Autodesk Fusion 360 part; units mm, degrees
(part 9 of 9)
  line L507 (94.532, 88.6913) -> (90.2019, 91.1913)
  line L508 (100.3622, 91.1913) -> (96.032, 88.6913)
  line L509 (96.032, 88.6913) -> (96.032, 83.6913)
  line L510 (96.032, 83.6913) -> (100.3622, 81.1913)
  line L511 (100.3622, 81.1913) -> (104.6923, 83.6913)
  line L512 (104.6923, 83.6913) -> (104.6923, 88.6913)
  line L513 (104.6923, 88.6913) -> (100.3622, 91.1913)
  line L514 (14, 99.9904) -> (9.6699, 97.4904)
  line L515 (9.6699, 97.4904) -> (9.6699, 92.4904)
  line L516 (9.6699, 92.4904) -> (14, 89.9904)
  line L517 (14, 89.9904) -> (18.3301, 92.4904)
  line L518 (18.3301, 92.4904) -> (18.3301, 97.4904)
  line L519 (18.3301, 97.4904) -> (14, 99.9904)
  line L520 (24.1603, 99.9904) -> (19.8301, 97.4904)
  line L521 (19.8301, 97.4904) -> (19.8301, 92.4904)
  line L522 (19.8301, 92.4904) -> (24.1603, 89.9904)
  line L523 (24.1603, 89.9904) -> (28.4904, 92.4904)
  line L524 (28.4904, 92.4904) -> (28.4904, 97.4904)
  line L525 (28.4904, 97.4904) -> (24.1603, 99.9904)
  line L526 (34.3205, 99.9904) -> (29.9904, 97.4904)
  line L527 (29.9904, 97.4904) -> (29.9904, 92.4904)
  line L528 (29.9904, 92.4904) -> (34.3205, 89.9904)
  line L529 (34.3205, 89.9904) -> (38.6506, 92.4904)
  line L530 (38.6506, 92.4904) -> (38.6506, 97.4904)
  line L531 (38.6506, 97.4904) -> (34.3205, 99.9904)
  line L532 (44.4808, 99.9904) -> (40.1506, 97.4904)
  line L533 (40.1506, 97.4904) -> (40.1506, 92.4904)
  line L534 (40.1506, 92.4904) -> (44.4808, 89.9904)
  line L535 (44.4808, 89.9904) -> (48.8109, 92.4904)
  line L536 (48.8109, 92.4904) -> (48.8109, 97.4904)
  line L537 (48.8109, 97.4904) -> (44.4808, 99.9904)
  line L538 (54.641, 99.9904) -> (50.3109, 97.4904)
  line L539 (50.3109, 97.4904) -> (50.3109, 92.4904)
  line L540 (50.3109, 92.4904) -> (54.641, 89.9904)
  line L541 (54.641, 89.9904) -> (58.9711, 92.4904)
  line L542 (58.9711, 92.4904) -> (58.9711, 97.4904)
  line L543 (58.9711, 97.4904) -> (54.641, 99.9904)
  line L544 (64.8013, 99.9904) -> (60.4711, 97.4904)
  line L545 (60.4711, 97.4904) -> (60.4711, 92.4904)
  line L546 (60.4711, 92.4904) -> (64.8013, 89.9904)
  line L547 (64.8013, 89.9904) -> (69.1314, 92.4904)
  line L548 (69.1314, 92.4904) -> (69.1314, 97.4904)
  line L549 (69.1314, 97.4904) -> (64.8013, 99.9904)
  line L550 (74.9615, 99.9904) -> (70.6314, 97.4904)
  line L551 (70.6314, 97.4904) -> (70.6314, 92.4904)
  line L552 (70.6314, 92.4904) -> (74.9615, 89.9904)
  line L553 (74.9615, 89.9904) -> (79.2916, 92.4904)
  line L554 (79.2916, 92.4904) -> (79.2916, 97.4904)
  line L555 (79.2916, 97.4904) -> (74.9615, 99.9904)
  line L556 (85.1218, 99.9904) -> (80.7916, 97.4904)
  line L557 (80.7916, 97.4904) -> (80.7916, 92.4904)
  line L558 (80.7916, 92.4904) -> (85.1218, 89.9904)
  line L559 (85.1218, 89.9904) -> (89.4519, 92.4904)
  line L560 (89.4519, 92.4904) -> (89.4519, 97.4904)
  line L561 (89.4519, 97.4904) -> (85.1218, 99.9904)
  line L562 (95.282, 99.9904) -> (90.9519, 97.4904)
  line L563 (90.9519, 97.4904) -> (90.9519, 92.4904)
  line L564 (90.9519, 92.4904) -> (95.282, 89.9904)
  line L565 (95.282, 89.9904) -> (99.6122, 92.4904)
  line L566 (99.6122, 92.4904) -> (99.6122, 97.4904)
  line L567 (99.6122, 97.4904) -> (95.282, 99.9904)
  line L568 (105.4423, 99.9904) -> (101.1122, 97.4904)
  line L569 (101.1122, 97.4904) -> (101.1122, 92.4904)
  line L570 (101.1122, 92.4904) -> (105.4423, 89.9904)
  line L571 (105.4423, 89.9904) -> (109.7724, 92.4904)
  line L572 (109.7724, 92.4904) -> (109.7724, 97.4904)
  line L573 (109.7724, 97.4904) -> (105.4423, 99.9904)
  line L574 (19.0801, 108.7894) -> (14.75, 106.2894)
  line L575 (14.75, 106.2894) -> (14.75, 101.2894)
  line L576 (14.75, 101.2894) -> (19.0801, 98.7894)
  line L577 (19.0801, 98.7894) -> (23.4103, 101.2894)
  line L578 (23.4103, 101.2894) -> (23.4103, 106.2894)
  line L579 (23.4103, 106.2894) -> (19.0801, 108.7894)
  line L580 (29.2404, 108.7894) -> (24.9103, 106.2894)
  line L581 (24.9103, 106.2894) -> (24.9103, 101.2894)
  line L582 (24.9103, 101.2894) -> (29.2404, 98.7894)
  line L583 (29.2404, 98.7894) -> (33.5705, 101.2894)
  line L584 (33.5705, 101.2894) -> (33.5705, 106.2894)
  line L585 (33.5705, 106.2894) -> (29.2404, 108.7894)
  line L586 (39.4006, 108.7894) -> (35.0705, 106.2894)
  line L587 (35.0705, 106.2894) -> (35.0705, 101.2894)
  line L588 (35.0705, 101.2894) -> (39.4006, 98.7894)
  line L589 (39.4006, 98.7894) -> (43.7308, 101.2894)
  line L590 (43.7308, 101.2894) -> (43.7308, 106.2894)
  line L591 (43.7308, 106.2894) -> (39.4006, 108.7894)
  line L592 (49.5609, 108.7894) -> (45.2308, 106.2894)
  line L593 (45.2308, 106.2894) -> (45.2308, 101.2894)
  line L594 (45.2308, 101.2894) -> (49.5609, 98.7894)
  line L595 (49.5609, 98.7894) -> (53.891, 101.2894)
  line L596 (53.891, 101.2894) -> (53.891, 106.2894)
  line L597 (53.891, 106.2894) -> (49.5609, 108.7894)
  line L598 (59.7211, 108.7894) -> (55.391, 106.2894)
  line L599 (55.391, 106.2894) -> (55.391, 101.2894)
  line L600 (55.391, 101.2894) -> (59.7211, 98.7894)
  line L601 (59.7211, 98.7894) -> (64.0513, 101.2894)
  line L602 (64.0513, 101.2894) -> (64.0513, 106.2894)
  line L603 (64.0513, 106.2894) -> (59.7211, 108.7894)
  line L604 (69.8814, 108.7894) -> (65.5513, 106.2894)
  line L605 (65.5513, 106.2894) -> (65.5513, 101.2894)
  line L606 (65.5513, 101.2894) -> (69.8814, 98.7894)
  line L607 (69.8814, 98.7894) -> (74.2115, 101.2894)
  line L608 (74.2115, 101.2894) -> (74.2115, 106.2894)
  line L609 (74.2115, 106.2894) -> (69.8814, 108.7894)
  line L610 (80.0416, 108.7894) -> (75.7115, 106.2894)
  line L611 (75.7115, 106.2894) -> (75.7115, 101.2894)
  line L612 (75.7115, 101.2894) -> (80.0416, 98.7894)
  line L613 (80.0416, 98.7894) -> (84.3718, 101.2894)
  line L614 (84.3718, 101.2894) -> (84.3718, 106.2894)
  line L615 (84.3718, 106.2894) -> (80.0416, 108.7894)
  line L616 (90.2019, 108.7894) -> (85.8718, 106.2894)
  line L617 (85.8718, 106.2894) -> (85.8718, 101.2894)
  line L618 (85.8718, 101.2894) -> (90.2019, 98.7894)
  line L619 (90.2019, 98.7894) -> (94.532, 101.2894)
  line L620 (94.532, 101.2894) -> (94.532, 106.2894)
  line L621 (94.532, 106.2894) -> (90.2019, 108.7894)
  line L622 (100.3622, 108.7894) -> (96.032, 106.2894)
  line L623 (96.032, 106.2894) -> (96.032, 101.2894)
  line L624 (96.032, 101.2894) -> (100.3622, 98.7894)
  line L625 (100.3622, 98.7894) -> (104.6923, 101.2894)
  line L626 (104.6923, 101.2894) -> (104.6923, 106.2894)
  line L627 (104.6923, 106.2894) -> (100.3622, 108.7894)
  line L628 (14, 117.5885) -> (9.6699, 115.0885)
  line L629 (9.6699, 115.0885) -> (9.6699, 110.0885)
  line L630 (9.6699, 110.0885) -> (14, 107.5885)
  line L631 (14, 107.5885) -> (18.3301, 110.0885)
  line L632 (18.3301, 110.0885) -> (18.3301, 115.0885)
  line L633 (18.3301, 115.0885) -> (14, 117.5885)
  line L634 (24.1603, 117.5885) -> (19.8301, 115.0885)
  line L635 (19.8301, 115.0885) -> (19.8301, 110.0885)
  line L636 (19.8301, 110.0885) -> (24.1603, 107.5885)
  line L637 (24.1603, 107.5885) -> (28.4904, 110.0885)
  line L638 (28.4904, 110.0885) -> (28.4904, 115.0885)
  line L639 (28.4904, 115.0885) -> (24.1603, 117.5885)
  line L640 (34.3205, 117.5885) -> (29.9904, 115.0885)
  line L641 (29.9904, 115.0885) -> (29.9904, 110.0885)
  line L642 (29.9904, 110.0885) -> (34.3205, 107.5885)
  line L643 (34.3205, 107.5885) -> (38.6506, 110.0885)
  line L644 (38.6506, 110.0885) -> (38.6506, 115.0885)
  line L645 (38.6506, 115.0885) -> (34.3205, 117.5885)
  line L646 (44.4808, 117.5885) -> (40.1506, 115.0885)
  line L647 (40.1506, 115.0885) -> (40.1506, 110.0885)
  line L648 (40.1506, 110.0885) -> (44.4808, 107.5885)
  line L649 (44.4808, 107.5885) -> (48.8109, 110.0885)
  line L650 (48.8109, 110.0885) -> (48.8109, 115.0885)
  line L651 (48.8109, 115.0885) -> (44.4808, 117.5885)
  line L652 (54.641, 117.5885) -> (50.3109, 115.0885)
  line L653 (50.3109, 115.0885) -> (50.3109, 110.0885)
  line L654 (50.3109, 110.0885) -> (54.641, 107.5885)
  line L655 (54.641, 107.5885) -> (58.9711, 110.0885)
  line L656 (58.9711, 110.0885) -> (58.9711, 115.0885)
  line L657 (58.9711, 115.0885) -> (54.641, 117.5885)
  line L658 (64.8013, 117.5885) -> (60.4711, 115.0885)
  line L659 (60.4711, 115.0885) -> (60.4711, 110.0885)
  line L660 (60.4711, 110.0885) -> (64.8013, 107.5885)
  line L661 (64.8013, 107.5885) -> (69.1314, 110.0885)
  line L662 (69.1314, 110.0885) -> (69.1314, 115.0885)
  line L663 (69.1314, 115.0885) -> (64.8013, 117.5885)
  line L664 (74.9615, 117.5885) -> (70.6314, 115.0885)
  line L665 (70.6314, 115.0885) -> (70.6314, 110.0885)
  line L666 (70.6314, 110.0885) -> (74.9615, 107.5885)
  line L667 (74.9615, 107.5885) -> (79.2916, 110.0885)
  line L668 (79.2916, 110.0885) -> (79.2916, 115.0885)
  line L669 (79.2916, 115.0885) -> (74.9615, 117.5885)
  line L670 (85.1218, 117.5885) -> (80.7916, 115.0885)
  line L671 (80.7916, 115.0885) -> (80.7916, 110.0885)
  line L672 (80.7916, 110.0885) -> (85.1218, 107.5885)
  line L673 (85.1218, 107.5885) -> (89.4519, 110.0885)
  line L674 (89.4519, 110.0885) -> (89.4519, 115.0885)
  line L675 (89.4519, 115.0885) -> (85.1218, 117.5885)
  line L676 (95.282, 117.5885) -> (90.9519, 115.0885)
  line L677 (90.9519, 115.0885) -> (90.9519, 110.0885)
  line L678 (90.9519, 110.0885) -> (95.282, 107.5885)
  line L679 (95.282, 107.5885) -> (99.6122, 110.0885)
  line L680 (99.6122, 110.0885) -> (99.6122, 115.0885)
  line L681 (99.6122, 115.0885) -> (95.282, 117.5885)
  line L682 (105.4423, 117.5885) -> (101.1122, 115.0885)
  line L683 (101.1122, 115.0885) -> (101.1122, 110.0885)
  line L684 (101.1122, 110.0885) -> (105.4423, 107.5885)
  line L685 (105.4423, 107.5885) -> (109.7724, 110.0885)
  line L686 (109.7724, 110.0885) -> (109.7724, 115.0885)
  line L687 (109.7724, 115.0885) -> (105.4423, 117.5885)
extrude "拉伸27" cut sketch "草图27" against normal blind 5 contours L4 L5 L6 L7 L8 L9 | L10 L11 L12 L13 L14 L15 | L16 L17 L18 L19 L20 L21 | L22 L23 L24 L25 L26 L27 | L28 L29 L30 L31 L32 L33 | L34 L35 L36 L37 L38 L39 | L40 L41 L42 L43 L44 L45 | L46 L47 L48 L49 L50 L51 | L52 L53 L54 L55 L56 L57 | L58 L59 L60 L61 L62 L63 | L64 L65 L66 L67 L68 L69 | L70 L71 L72 L73 L74 L75 | L76 L77 L78 L79 L80 L81 | L82 L83 L84 L85 L86 L87 | L88 L89 L90 L91 L92 L93 | L94 L95 L96 L97 L98 L99 | L100 L101 L102 L103 L104 L105 | L106 L107 L108 L109 L110 L111 | L112 L113 L114 L115 L116 L117 | L118 L119 L120 L121 L122 L123 | L124 L125 L126 L127 L128 L129 | L130 L131 L132 L133 L134 L135 | L136 L137 L138 L139 L140 L141 | L142 L143 L144 L145 L146 L147 | L148 L149 L150 L151 L152 L153 | L154 L155 L156 L157 L158 L159 | L160 L161 L162 L163 L164 L165 | L166 L167 L168 L169 L170 L171 | L172 L173 L174 L175 L176 L177 | L178 L179 L180 L181 L182 L183 | L184 L185 L186 L187 L188 L189 | L190 L191 L192 L193 L194 L195 | L196 L197 L198 L199 L200 L201 | L202 L203 L204 L205 L206 L207 | L208 L209 L210 L211 L212 L213 | L214 L215 L216 L217 L218 L219 | L220 L221 L222 L223 L224 L225 | L226 L227 L228 L229 L230 L231 | L232 L233 L234 L235 L236 L237 | L238 L239 L240 L241 L242 L243 | L244 L245 L246 L247 L248 L249 | L250 L251 L252 L253 L254 L255 | L256 L257 L258 L259 L260 L261 | L262 L263 L264 L265 L266 L267 | L268 L269 L270 L271 L272 L273 | L274 L275 L276 L277 L278 L279 | L280 L281 L282 L283 L284 L285 | L286 L287 L288 L289 L290 L291 | L292 L293 L294 L295 L296 L297 | L298 L299 L300 L301 L302 L303 | L304 L305 L306 L307 L308 L309 | L310 L311 L312 L313 L314 L315 | L316 L317 L318 L319 L320 L321 | L322 L323 L324 L325 L326 L327 | L328 L329 L330 L331 L332 L333 | L334 L335 L336 L337 L338 L339 | L340 L341 L342 L343 L344 L345 | L346 L347 L348 L349 L350 L351 | L352 L353 L354 L355 L356 L357 | L358 L359 L360 L361 L362 L363 | L364 L365 L366 L367 L368 L369 | L370 L371 L372 L373 L374 L375 | L376 L377 L378 L379 L380 L381 | L382 L383 L384 L385 L386 L387 | L388 L389 L390 L391 L392 L393 | L394 L395 L396 L397 L398 L399 | L400 L401 L402 L403 L404 L405 | L406 L407 L408 L409 L410 L411 | L412 L413 L414 L415 L416 L417 | L418 L419 L420 L421 L422 L423 | L424 L425 L426 L427 L428 L429 | L430 L431 L432 L433 L434 L435 | L436 L437 L438 L439 L440 L441 | L442 L443 L444 L445 L446 L447 | L448 L449 L450 L451 L452 L453 | L454 L455 L456 L457 L458 L459 | L460 L461 L462 L463 L464 L465 | L466 L467 L468 L469 L470 L471 | L472 L473 L474 L475 L476 L477 | L478 L479 L480 L481 L482 L483 | L484 L485 L486 L487 L488 L489 | L490 L491 L492 L493 L494 L495 | L496 L497 L498 L499 L500 L501 | L502 L503 L504 L505 L506 L507 | L508 L509 L510 L511 L512 L513 | L514 L515 L516 L517 L518 L519 | L520 L521 L522 L523 L524 L525 | L526 L527 L528 L529 L530 L531 | L532 L533 L534 L535 L536 L537 | L538 L539 L540 L541 L542 L543 | L544 L545 L546 L547 L548 L549 | L550 L551 L552 L553 L554 L555 | L556 L557 L558 L559 L560 L561 | L562 L563 L564 L565 L566 L567 | L568 L569 L570 L571 L572 L573 | L574 L575 L576 L577 L578 L579 | L580 L581 L582 L583 L584 L585 | L586 L587 L588 L589 L590 L591 | L592 L593 L594 L595 L596 L597 | L598 L599 L600 L601 L602 L603 | L604 L605 L606 L607 L608 L609 | L610 L611 L612 L613 L614 L615 | L616 L617 L618 L619 L620 L621 | L622 L623 L624 L625 L626 L627 | L628 L629 L630 L631 L632 L633 | L634 L635 L636 L637 L638 L639 | L640 L641 L642 L643 L644 L645 | L646 L647 L648 L649 L650 L651 | L652 L653 L654 L655 L656 L657 | L658 L659 L660 L661 L662 L663 | L664 L665 L666 L667 L668 L669 | L670 L671 L672 L673 L674 L675 | L676 L677 L678 L679 L680 L681 | L682 L683 L684 L685 L686 L687 bodies 1 4
sketch "草图28" plane through (0, 116, 0) normal (0, -1, 0) x (1, 0, 0)
  line L0 (7, 0) -> (69, 0)
  line L1 (69, 0) -> (69, 90)
  line L2 (69, 90) -> (7, 90)
  line L3 (7, 90) -> (7, 65)
  line L4 (7, 65) -> (7, 0)
  line L5 (19.3301, 21.2321) -> (15, 18.7321)
  line L6 (15, 18.7321) -> (15, 13.7321)
  line L7 (15, 13.7321) -> (19.3301, 11.2321)
  line L8 (19.3301, 11.2321) -> (23.6603, 13.7321)
  line L9 (23.6603, 13.7321) -> (23.6603, 18.7321)
  line L10 (23.6603, 18.7321) -> (19.3301, 21.2321)
  line L11 (29.9904, 21.2321) -> (25.6603, 18.7321)
  line L12 (25.6603, 18.7321) -> (25.6603, 13.7321)
  line L13 (25.6603, 13.7321) -> (29.9904, 11.2321)
  line L14 (29.9904, 11.2321) -> (34.3205, 13.7321)
  line L15 (34.3205, 13.7321) -> (34.3205, 18.7321)
  line L16 (34.3205, 18.7321) -> (29.9904, 21.2321)
  line L17 (40.6506, 21.2321) -> (36.3205, 18.7321)
  line L18 (36.3205, 18.7321) -> (36.3205, 13.7321)
  line L19 (36.3205, 13.7321) -> (40.6506, 11.2321)
  line L20 (40.6506, 11.2321) -> (44.9808, 13.7321)
  line L21 (44.9808, 13.7321) -> (44.9808, 18.7321)
  line L22 (44.9808, 18.7321) -> (40.6506, 21.2321)
  line L23 (51.3109, 21.2321) -> (46.9808, 18.7321)
  line L24 (46.9808, 18.7321) -> (46.9808, 13.7321)
  line L25 (46.9808, 13.7321) -> (51.3109, 11.2321)
  line L26 (51.3109, 11.2321) -> (55.641, 13.7321)
  line L27 (55.641, 13.7321) -> (55.641, 18.7321)
  line L28 (55.641, 18.7321) -> (51.3109, 21.2321)
  line L29 (61.9711, 21.2321) -> (57.641, 18.7321)
  line L30 (57.641, 18.7321) -> (57.641, 13.7321)
  line L31 (57.641, 13.7321) -> (61.9711, 11.2321)
  line L32 (61.9711, 11.2321) -> (66.3013, 13.7321)
  line L33 (66.3013, 13.7321) -> (66.3013, 18.7321)
  line L34 (66.3013, 18.7321) -> (61.9711, 21.2321)
  line L35 (14, 30.4641) -> (9.6699, 27.9641)
  line L36 (9.6699, 27.9641) -> (9.6699, 22.9641)
  line L37 (9.6699, 22.9641) -> (14, 20.4641)
  line L38 (14, 20.4641) -> (18.3301, 22.9641)
  line L39 (18.3301, 22.9641) -> (18.3301, 27.9641)
  line L40 (18.3301, 27.9641) -> (14, 30.4641)
  line L41 (24.6603, 30.4641) -> (20.3301, 27.9641)
  line L42 (20.3301, 27.9641) -> (20.3301, 22.9641)
  line L43 (20.3301, 22.9641) -> (24.6603, 20.4641)
  line L44 (24.6603, 20.4641) -> (28.9904, 22.9641)
  line L45 (28.9904, 22.9641) -> (28.9904, 27.9641)
  line L46 (28.9904, 27.9641) -> (24.6603, 30.4641)
  line L47 (35.3205, 30.4641) -> (30.9904, 27.9641)
  line L48 (30.9904, 27.9641) -> (30.9904, 22.9641)
  line L49 (30.9904, 22.9641) -> (35.3205, 20.4641)
  line L50 (35.3205, 20.4641) -> (39.6506, 22.9641)
  line L51 (39.6506, 22.9641) -> (39.6506, 27.9641)
  line L52 (39.6506, 27.9641) -> (35.3205, 30.4641)
  line L53 (45.9808, 30.4641) -> (41.6506, 27.9641)
  line L54 (41.6506, 27.9641) -> (41.6506, 22.9641)
  line L55 (41.6506, 22.9641) -> (45.9808, 20.4641)
  line L56 (45.9808, 20.4641) -> (50.3109, 22.9641)
  line L57 (50.3109, 22.9641) -> (50.3109, 27.9641)
  line L58 (50.3109, 27.9641) -> (45.9808, 30.4641)
  line L59 (56.641, 30.4641) -> (52.3109, 27.9641)
  line L60 (52.3109, 27.9641) -> (52.3109, 22.9641)
  line L61 (52.3109, 22.9641) -> (56.641, 20.4641)
  line L62 (56.641, 20.4641) -> (60.9711, 22.9641)
  line L63 (60.9711, 22.9641) -> (60.9711, 27.9641)
  line L64 (60.9711, 27.9641) -> (56.641, 30.4641)
  line L65 (19.3301, 39.6962) -> (15, 37.1962)
  line L66 (15, 37.1962) -> (15, 32.1962)
  line L67 (15, 32.1962) -> (19.3301, 29.6962)
  line L68 (19.3301, 29.6962) -> (23.6603, 32.1962)
  line L69 (23.6603, 32.1962) -> (23.6603, 37.1962)
  line L70 (23.6603, 37.1962) -> (19.3301, 39.6962)
  line L71 (29.9904, 39.6962) -> (25.6603, 37.1962)
  line L72 (25.6603, 37.1962) -> (25.6603, 32.1962)
  line L73 (25.6603, 32.1962) -> (29.9904, 29.6962)
  line L74 (29.9904, 29.6962) -> (34.3205, 32.1962)
  line L75 (34.3205, 32.1962) -> (34.3205, 37.1962)
  line L76 (34.3205, 37.1962) -> (29.9904, 39.6962)
  line L77 (40.6506, 39.6962) -> (36.3205, 37.1962)
  line L78 (36.3205, 37.1962) -> (36.3205, 32.1962)
  line L79 (36.3205, 32.1962) -> (40.6506, 29.6962)
  line L80 (40.6506, 29.6962) -> (44.9808, 32.1962)
  line L81 (44.9808, 32.1962) -> (44.9808, 37.1962)
  line L82 (44.9808, 37.1962) -> (40.6506, 39.6962)
  line L83 (51.3109, 39.6962) -> (46.9808, 37.1962)
  line L84 (46.9808, 37.1962) -> (46.9808, 32.1962)
  line L85 (46.9808, 32.1962) -> (51.3109, 29.6962)
  line L86 (51.3109, 29.6962) -> (55.641, 32.1962)
  line L87 (55.641, 32.1962) -> (55.641, 37.1962)
  line L88 (55.641, 37.1962) -> (51.3109, 39.6962)
  line L89 (61.9711, 39.6962) -> (57.641, 37.1962)
  line L90 (57.641, 37.1962) -> (57.641, 32.1962)
  line L91 (57.641, 32.1962) -> (61.9711, 29.6962)
  line L92 (61.9711, 29.6962) -> (66.3013, 32.1962)
  line L93 (66.3013, 32.1962) -> (66.3013, 37.1962)
  line L94 (66.3013, 37.1962) -> (61.9711, 39.6962)
  line L95 (14, 48.9282) -> (9.6699, 46.4282)
  line L96 (9.6699, 46.4282) -> (9.6699, 41.4282)
  line L97 (9.6699, 41.4282) -> (14, 38.9282)
  line L98 (14, 38.9282) -> (18.3301, 41.4282)
  line L99 (18.3301, 41.4282) -> (18.3301, 46.4282)
  line L100 (18.3301, 46.4282) -> (14, 48.9282)
  line L101 (24.6603, 48.9282) -> (20.3301, 46.4282)
  line L102 (20.3301, 46.4282) -> (20.3301, 41.4282)
  line L103 (20.3301, 41.4282) -> (24.6603, 38.9282)
  line L104 (24.6603, 38.9282) -> (28.9904, 41.4282)
  line L105 (28.9904, 41.4282) -> (28.9904, 46.4282)
  line L106 (28.9904, 46.4282) -> (24.6603, 48.9282)
  line L107 (35.3205, 48.9282) -> (30.9904, 46.4282)
  line L108 (30.9904, 46.4282) -> (30.9904, 41.4282)
  line L109 (30.9904, 41.4282) -> (35.3205, 38.9282)
  line L110 (35.3205, 38.9282) -> (39.6506, 41.4282)
  line L111 (39.6506, 41.4282) -> (39.6506, 46.4282)
  line L112 (39.6506, 46.4282) -> (35.3205, 48.9282)
  line L113 (45.9808, 48.9282) -> (41.6506, 46.4282)
  line L114 (41.6506, 46.4282) -> (41.6506, 41.4282)
  line L115 (41.6506, 41.4282) -> (45.9808, 38.9282)
  line L116 (45.9808, 38.9282) -> (50.3109, 41.4282)
  line L117 (50.3109, 41.4282) -> (50.3109, 46.4282)
  line L118 (50.3109, 46.4282) -> (45.9808, 48.9282)
  line L119 (56.641, 48.9282) -> (52.3109, 46.4282)
  line L120 (52.3109, 46.4282) -> (52.3109, 41.4282)
  line L121 (52.3109, 41.4282) -> (56.641, 38.9282)
  line L122 (56.641, 38.9282) -> (60.9711, 41.4282)
  line L123 (60.9711, 41.4282) -> (60.9711, 46.4282)
  line L124 (60.9711, 46.4282) -> (56.641, 48.9282)
  line L125 (19.3301, 58.1603) -> (15, 55.6603)
  line L126 (15, 55.6603) -> (15, 50.6603)
  line L127 (15, 50.6603) -> (19.3301, 48.1603)
  line L128 (19.3301, 48.1603) -> (23.6603, 50.6603)
  line L129 (23.6603, 50.6603) -> (23.6603, 55.6603)
  line L130 (23.6603, 55.6603) -> (19.3301, 58.1603)
  line L131 (29.9904, 58.1603) -> (25.6603, 55.6603)
  line L132 (25.6603, 55.6603) -> (25.6603, 50.6603)
  line L133 (25.6603, 50.6603) -> (29.9904, 48.1603)
  line L134 (29.9904, 48.1603) -> (34.3205, 50.6603)
  line L135 (34.3205, 50.6603) -> (34.3205, 55.6603)
  line L136 (34.3205, 55.6603) -> (29.9904, 58.1603)
  line L137 (40.6506, 58.1603) -> (36.3205, 55.6603)
  line L138 (36.3205, 55.6603) -> (36.3205, 50.6603)
  line L139 (36.3205, 50.6603) -> (40.6506, 48.1603)
  line L140 (40.6506, 48.1603) -> (44.9808, 50.6603)
  line L141 (44.9808, 50.6603) -> (44.9808, 55.6603)
  line L142 (44.9808, 55.6603) -> (40.6506, 58.1603)
  line L143 (51.3109, 58.1603) -> (46.9808, 55.6603)
  line L144 (46.9808, 55.6603) -> (46.9808, 50.6603)
  line L145 (46.9808, 50.6603) -> (51.3109, 48.1603)
  line L146 (51.3109, 48.1603) -> (55.641, 50.6603)
  line L147 (55.641, 50.6603) -> (55.641, 55.6603)
  line L148 (55.641, 55.6603) -> (51.3109, 58.1603)
  line L149 (61.9711, 58.1603) -> (57.641, 55.6603)
  line L150 (57.641, 55.6603) -> (57.641, 50.6603)
  line L151 (57.641, 50.6603) -> (61.9711, 48.1603)
  line L152 (61.9711, 48.1603) -> (66.3013, 50.6603)
  line L153 (66.3013, 50.6603) -> (66.3013, 55.6603)
  line L154 (66.3013, 55.6603) -> (61.9711, 58.1603)
  line L155 (14, 67.3923) -> (9.6699, 64.8923)
  line L156 (9.6699, 64.8923) -> (9.6699, 59.8923)
  line L157 (9.6699, 59.8923) -> (14, 57.3923)
  line L158 (14, 57.3923) -> (18.3301, 59.8923)
  line L159 (18.3301, 59.8923) -> (18.3301, 64.8923)
  line L160 (18.3301, 64.8923) -> (14, 67.3923)
  line L161 (24.6603, 67.3923) -> (20.3301, 64.8923)
  line L162 (20.3301, 64.8923) -> (20.3301, 59.8923)
  line L163 (20.3301, 59.8923) -> (24.6603, 57.3923)
  line L164 (24.6603, 57.3923) -> (28.9904, 59.8923)
  line L165 (28.9904, 59.8923) -> (28.9904, 64.8923)
  line L166 (28.9904, 64.8923) -> (24.6603, 67.3923)
  line L167 (35.3205, 67.3923) -> (30.9904, 64.8923)
  line L168 (30.9904, 64.8923) -> (30.9904, 59.8923)
  line L169 (30.9904, 59.8923) -> (35.3205, 57.3923)
  line L170 (35.3205, 57.3923) -> (39.6506, 59.8923)
  line L171 (39.6506, 59.8923) -> (39.6506, 64.8923)
  line L172 (39.6506, 64.8923) -> (35.3205, 67.3923)
  line L173 (45.9808, 67.3923) -> (41.6506, 64.8923)
  line L174 (41.6506, 64.8923) -> (41.6506, 59.8923)
  line L175 (41.6506, 59.8923) -> (45.9808, 57.3923)
  line L176 (45.9808, 57.3923) -> (50.3109, 59.8923)
  line L177 (50.3109, 59.8923) -> (50.3109, 64.8923)
  line L178 (50.3109, 64.8923) -> (45.9808, 67.3923)
  line L179 (56.641, 67.3923) -> (52.3109, 64.8923)
  line L180 (52.3109, 64.8923) -> (52.3109, 59.8923)
  line L181 (52.3109, 59.8923) -> (56.641, 57.3923)
  line L182 (56.641, 57.3923) -> (60.9711, 59.8923)
  line L183 (60.9711, 59.8923) -> (60.9711, 64.8923)
  line L184 (60.9711, 64.8923) -> (56.641, 67.3923)
  line L185 (19.3301, 76.6244) -> (15, 74.1244)
  line L186 (15, 74.1244) -> (15, 69.1244)
  line L187 (15, 69.1244) -> (19.3301, 66.6244)
  line L188 (19.3301, 66.6244) -> (23.6603, 69.1244)
  line L189 (23.6603, 69.1244) -> (23.6603, 74.1244)
  line L190 (23.6603, 74.1244) -> (19.3301, 76.6244)
  line L191 (29.9904, 76.6244) -> (25.6603, 74.1244)
  line L192 (25.6603, 74.1244) -> (25.6603, 69.1244)
  line L193 (25.6603, 69.1244) -> (29.9904, 66.6244)
  line L194 (29.9904, 66.6244) -> (34.3205, 69.1244)
  line L195 (34.3205, 69.1244) -> (34.3205, 74.1244)
  line L196 (34.3205, 74.1244) -> (29.9904, 76.6244)
  line L197 (40.6506, 76.6244) -> (36.3205, 74.1244)
  line L198 (36.3205, 74.1244) -> (36.3205, 69.1244)
  line L199 (36.3205, 69.1244) -> (40.6506, 66.6244)
  line L200 (40.6506, 66.6244) -> (44.9808, 69.1244)
  line L201 (44.9808, 69.1244) -> (44.9808, 74.1244)
  line L202 (44.9808, 74.1244) -> (40.6506, 76.6244)
  line L203 (51.3109, 76.6244) -> (46.9808, 74.1244)
  line L204 (46.9808, 74.1244) -> (46.9808, 69.1244)
  line L205 (46.9808, 69.1244) -> (51.3109, 66.6244)
  line L206 (51.3109, 66.6244) -> (55.641, 69.1244)
  line L207 (55.641, 69.1244) -> (55.641, 74.1244)
  line L208 (55.641, 74.1244) -> (51.3109, 76.6244)
  line L209 (61.9711, 76.6244) -> (57.641, 74.1244)
  line L210 (57.641, 74.1244) -> (57.641, 69.1244)
  line L211 (57.641, 69.1244) -> (61.9711, 66.6244)
  line L212 (61.9711, 66.6244) -> (66.3013, 69.1244)
  line L213 (66.3013, 69.1244) -> (66.3013, 74.1244)
  line L214 (66.3013, 74.1244) -> (61.9711, 76.6244)
  line L215 (14, 85.8564) -> (9.6699, 83.3564)
  line L216 (9.6699, 83.3564) -> (9.6699, 78.3564)
  line L217 (9.6699, 78.3564) -> (14, 75.8564)
  line L218 (14, 75.8564) -> (18.3301, 78.3564)
  line L219 (18.3301, 78.3564) -> (18.3301, 83.3564)
  line L220 (18.3301, 83.3564) -> (14, 85.8564)
  line L221 (24.6603, 85.8564) -> (20.3301, 83.3564)
  line L222 (20.3301, 83.3564) -> (20.3301, 78.3564)
  line L223 (20.3301, 78.3564) -> (24.6603, 75.8564)
  line L224 (24.6603, 75.8564) -> (28.9904, 78.3564)
  line L225 (28.9904, 78.3564) -> (28.9904, 83.3564)
  line L226 (28.9904, 83.3564) -> (24.6603, 85.8564)
  line L227 (35.3205, 85.8564) -> (30.9904, 83.3564)
  line L228 (30.9904, 83.3564) -> (30.9904, 78.3564)
  line L229 (30.9904, 78.3564) -> (35.3205, 75.8564)
  line L230 (35.3205, 75.8564) -> (39.6506, 78.3564)
  line L231 (39.6506, 78.3564) -> (39.6506, 83.3564)
  line L232 (39.6506, 83.3564) -> (35.3205, 85.8564)
  line L233 (45.9808, 85.8564) -> (41.6506, 83.3564)
  line L234 (41.6506, 83.3564) -> (41.6506, 78.3564)
  line L235 (41.6506, 78.3564) -> (45.9808, 75.8564)
  line L236 (45.9808, 75.8564) -> (50.3109, 78.3564)
  line L237 (50.3109, 78.3564) -> (50.3109, 83.3564)
  line L238 (50.3109, 83.3564) -> (45.9808, 85.8564)
  line L239 (56.641, 85.8564) -> (52.3109, 83.3564)
  line L240 (52.3109, 83.3564) -> (52.3109, 78.3564)
  line L241 (52.3109, 78.3564) -> (56.641, 75.8564)
  line L242 (56.641, 75.8564) -> (60.9711, 78.3564)
  line L243 (60.9711, 78.3564) -> (60.9711, 83.3564)
  line L244 (60.9711, 83.3564) -> (56.641, 85.8564)
extrude "拉伸28" cut sketch "草图28" against normal blind 5 contours L5 L6 L7 L8 L9 L10 | L11 L12 L13 L14 L15 L16 | L17 L18 L19 L20 L21 L22 | L23 L24 L25 L26 L27 L28 | L29 L30 L31 L32 L33 L34 | L35 L36 L37 L38 L39 L40 | L41 L42 L43 L44 L45 L46 | L47 L48 L49 L50 L51 L52 | L53 L54 L55 L56 L57 L58 | L59 L60 L61 L62 L63 L64 | L65 L66 L67 L68 L69 L70 | L71 L72 L73 L74 L75 L76 | L77 L78 L79 L80 L81 L82 | L83 L84 L85 L86 L87 L88 | L89 L90 L91 L92 L93 L94 | L95 L96 L97 L98 L99 L100 | L101 L102 L103 L104 L105 L106 | L107 L108 L109 L110 L111 L112 | L113 L114 L115 L116 L117 L118 | L119 L120 L121 L122 L123 L124 | L125 L126 L127 L128 L129 L130 | L131 L132 L133 L134 L135 L136 | L137 L138 L139 L140 L141 L142 | L143 L144 L145 L146 L147 L148 | L149 L150 L151 L152 L153 L154 | L155 L156 L157 L158 L159 L160 | L161 L162 L163 L164 L165 L166 | L167 L168 L169 L170 L171 L172 | L173 L174 L175 L176 L177 L178 | L179 L180 L181 L182 L183 L184 | L185 L186 L187 L188 L189 L190 | L191 L192 L193 L194 L195 L196 | L197 L198 L199 L200 L201 L202 | L203 L204 L205 L206 L207 L208 | L209 L210 L211 L212 L213 L214 | L215 L216 L217 L218 L219 L220 | L221 L222 L223 L224 L225 L226 | L227 L228 L229 L230 L231 L232 | L233 L234 L235 L236 L237 L238 | L239 L240 L241 L242 L243 L244 bodies 1
sketch "草图29" plane through (0, 116, 0) normal (0, -1, 0) x (1, 0, 0)
  line L0 (72, 0) -> (116, 0)
  line L1 (116, 0) -> (116, 140)
  line L2 (116, 140) -> (72, 140)
  line L3 (72, 140) -> (72, 65)
  line L4 (72, 65) -> (72, 0)
  line L5 (84.3301, 21.2321) -> (80, 18.7321)
  line L6 (80, 18.7321) -> (80, 13.7321)
  line L7 (80, 13.7321) -> (84.3301, 11.2321)
  line L8 (84.3301, 11.2321) -> (88.6603, 13.7321)
  line L9 (88.6603, 13.7321) -> (88.6603, 18.7321)
  line L10 (88.6603, 18.7321) -> (84.3301, 21.2321)
  line L11 (94.9904, 21.2321) -> (90.6603, 18.7321)
  line L12 (90.6603, 18.7321) -> (90.6603, 13.7321)
  line L13 (90.6603, 13.7321) -> (94.9904, 11.2321)
  line L14 (94.9904, 11.2321) -> (99.3205, 13.7321)
  line L15 (99.3205, 13.7321) -> (99.3205, 18.7321)
  line L16 (99.3205, 18.7321) -> (94.9904, 21.2321)
  line L17 (105.6506, 21.2321) -> (101.3205, 18.7321)
  line L18 (101.3205, 18.7321) -> (101.3205, 13.7321)
  line L19 (101.3205, 13.7321) -> (105.6506, 11.2321)
  line L20 (105.6506, 11.2321) -> (109.9808, 13.7321)
  line L21 (109.9808, 13.7321) -> (109.9808, 18.7321)
  line L22 (109.9808, 18.7321) -> (105.6506, 21.2321)
  line L23 (79, 30.4641) -> (74.6699, 27.9641)
  line L24 (74.6699, 27.9641) -> (74.6699, 22.9641)
  line L25 (74.6699, 22.9641) -> (79, 20.4641)
  line L26 (79, 20.4641) -> (83.3301, 22.9641)
  line L27 (83.3301, 22.9641) -> (83.3301, 27.9641)
  line L28 (83.3301, 27.9641) -> (79, 30.4641)
  line L29 (89.6603, 30.4641) -> (85.3301, 27.9641)
  line L30 (85.3301, 27.9641) -> (85.3301, 22.9641)
  line L31 (85.3301, 22.9641) -> (89.6603, 20.4641)
  line L32 (89.6603, 20.4641) -> (93.9904, 22.9641)
  line L33 (93.9904, 22.9641) -> (93.9904, 27.9641)
  line L34 (93.9904, 27.9641) -> (89.6603, 30.4641)
  line L35 (100.3205, 30.4641) -> (95.9904, 27.9641)
  line L36 (95.9904, 27.9641) -> (95.9904, 22.9641)
  line L37 (95.9904, 22.9641) -> (100.3205, 20.4641)
  line L38 (100.3205, 20.4641) -> (104.6506, 22.9641)
  line L39 (104.6506, 22.9641) -> (104.6506, 27.9641)
  line L40 (104.6506, 27.9641) -> (100.3205, 30.4641)
  line L41 (84.3301, 39.6962) -> (80, 37.1962)
  line L42 (80, 37.1962) -> (80, 32.1962)
  line L43 (80, 32.1962) -> (84.3301, 29.6962)
  line L44 (84.3301, 29.6962) -> (88.6603, 32.1962)
  line L45 (88.6603, 32.1962) -> (88.6603, 37.1962)
  line L46 (88.6603, 37.1962) -> (84.3301, 39.6962)
  line L47 (94.9904, 39.6962) -> (90.6603, 37.1962)
  line L48 (90.6603, 37.1962) -> (90.6603, 32.1962)
  line L49 (90.6603, 32.1962) -> (94.9904, 29.6962)
  line L50 (94.9904, 29.6962) -> (99.3205, 32.1962)
  line L51 (99.3205, 32.1962) -> (99.3205, 37.1962)
  line L52 (99.3205, 37.1962) -> (94.9904, 39.6962)
  line L53 (105.6506, 39.6962) -> (101.3205, 37.1962)
  line L54 (101.3205, 37.1962) -> (101.3205, 32.1962)
  line L55 (101.3205, 32.1962) -> (105.6506, 29.6962)
  line L56 (105.6506, 29.6962) -> (109.9808, 32.1962)
  line L57 (109.9808, 32.1962) -> (109.9808, 37.1962)
  line L58 (109.9808, 37.1962) -> (105.6506, 39.6962)
  line L59 (79, 48.9282) -> (74.6699, 46.4282)
  line L60 (74.6699, 46.4282) -> (74.6699, 41.4282)
  line L61 (74.6699, 41.4282) -> (79, 38.9282)
  line L62 (79, 38.9282) -> (83.3301, 41.4282)
  line L63 (83.3301, 41.4282) -> (83.3301, 46.4282)
  line L64 (83.3301, 46.4282) -> (79, 48.9282)
  line L65 (89.6603, 48.9282) -> (85.3301, 46.4282)
  line L66 (85.3301, 46.4282) -> (85.3301, 41.4282)
  line L67 (85.3301, 41.4282) -> (89.6603, 38.9282)
  line L68 (89.6603, 38.9282) -> (93.9904, 41.4282)
  line L69 (93.9904, 41.4282) -> (93.9904, 46.4282)
  line L70 (93.9904, 46.4282) -> (89.6603, 48.9282)
  line L71 (100.3205, 48.9282) -> (95.9904, 46.4282)
  line L72 (95.9904, 46.4282) -> (95.9904, 41.4282)
  line L73 (95.9904, 41.4282) -> (100.3205, 38.9282)
  line L74 (100.3205, 38.9282) -> (104.6506, 41.4282)
  line L75 (104.6506, 41.4282) -> (104.6506, 46.4282)
  line L76 (104.6506, 46.4282) -> (100.3205, 48.9282)
  line L77 (84.3301, 58.1603) -> (80, 55.6603)
  line L78 (80, 55.6603) -> (80, 50.6603)
  line L79 (80, 50.6603) -> (84.3301, 48.1603)
  line L80 (84.3301, 48.1603) -> (88.6603, 50.6603)
  line L81 (88.6603, 50.6603) -> (88.6603, 55.6603)
  line L82 (88.6603, 55.6603) -> (84.3301, 58.1603)
  line L83 (94.9904, 58.1603) -> (90.6603, 55.6603)
  line L84 (90.6603, 55.6603) -> (90.6603, 50.6603)
  line L85 (90.6603, 50.6603) -> (94.9904, 48.1603)
  line L86 (94.9904, 48.1603) -> (99.3205, 50.6603)
  line L87 (99.3205, 50.6603) -> (99.3205, 55.6603)
  line L88 (99.3205, 55.6603) -> (94.9904, 58.1603)
  line L89 (105.6506, 58.1603) -> (101.3205, 55.6603)
  line L90 (101.3205, 55.6603) -> (101.3205, 50.6603)
  line L91 (101.3205, 50.6603) -> (105.6506, 48.1603)
  line L92 (105.6506, 48.1603) -> (109.9808, 50.6603)
  line L93 (109.9808, 50.6603) -> (109.9808, 55.6603)
  line L94 (109.9808, 55.6603) -> (105.6506, 58.1603)
  line L95 (79, 67.3923) -> (74.6699, 64.8923)
  line L96 (74.6699, 64.8923) -> (74.6699, 59.8923)
  line L97 (74.6699, 59.8923) -> (79, 57.3923)
  line L98 (79, 57.3923) -> (83.3301, 59.8923)
  line L99 (83.3301, 59.8923) -> (83.3301, 64.8923)
  line L100 (83.3301, 64.8923) -> (79, 67.3923)
  line L101 (89.6603, 67.3923) -> (85.3301, 64.8923)
  line L102 (85.3301, 64.8923) -> (85.3301, 59.8923)
  line L103 (85.3301, 59.8923) -> (89.6603, 57.3923)
  line L104 (89.6603, 57.3923) -> (93.9904, 59.8923)
  line L105 (93.9904, 59.8923) -> (93.9904, 64.8923)
  line L106 (93.9904, 64.8923) -> (89.6603, 67.3923)
  line L107 (100.3205, 67.3923) -> (95.9904, 64.8923)
  line L108 (95.9904, 64.8923) -> (95.9904, 59.8923)
  line L109 (95.9904, 59.8923) -> (100.3205, 57.3923)
  line L110 (100.3205, 57.3923) -> (104.6506, 59.8923)
  line L111 (104.6506, 59.8923) -> (104.6506, 64.8923)
  line L112 (104.6506, 64.8923) -> (100.3205, 67.3923)
  line L113 (84.3301, 76.6244) -> (80, 74.1244)
  line L114 (80, 74.1244) -> (80, 69.1244)
  line L115 (80, 69.1244) -> (84.3301, 66.6244)
  line L116 (84.3301, 66.6244) -> (88.6603, 69.1244)
  line L117 (88.6603, 69.1244) -> (88.6603, 74.1244)
  line L118 (88.6603, 74.1244) -> (84.3301, 76.6244)
  line L119 (94.9904, 76.6244) -> (90.6603, 74.1244)
  line L120 (90.6603, 74.1244) -> (90.6603, 69.1244)
  line L121 (90.6603, 69.1244) -> (94.9904, 66.6244)
  line L122 (94.9904, 66.6244) -> (99.3205, 69.1244)
  line L123 (99.3205, 69.1244) -> (99.3205, 74.1244)
  line L124 (99.3205, 74.1244) -> (94.9904, 76.6244)
  line L125 (105.6506, 76.6244) -> (101.3205, 74.1244)
  line L126 (101.3205, 74.1244) -> (101.3205, 69.1244)
  line L127 (101.3205, 69.1244) -> (105.6506, 66.6244)
  line L128 (105.6506, 66.6244) -> (109.9808, 69.1244)
  line L129 (109.9808, 69.1244) -> (109.9808, 74.1244)
  line L130 (109.9808, 74.1244) -> (105.6506, 76.6244)
  line L131 (79, 85.8564) -> (74.6699, 83.3564)
  line L132 (74.6699, 83.3564) -> (74.6699, 78.3564)
  line L133 (74.6699, 78.3564) -> (79, 75.8564)
  line L134 (79, 75.8564) -> (83.3301, 78.3564)
  line L135 (83.3301, 78.3564) -> (83.3301, 83.3564)
  line L136 (83.3301, 83.3564) -> (79, 85.8564)
  line L137 (89.6603, 85.8564) -> (85.3301, 83.3564)
  line L138 (85.3301, 83.3564) -> (85.3301, 78.3564)
  line L139 (85.3301, 78.3564) -> (89.6603, 75.8564)
  line L140 (89.6603, 75.8564) -> (93.9904, 78.3564)
  line L141 (93.9904, 78.3564) -> (93.9904, 83.3564)
  line L142 (93.9904, 83.3564) -> (89.6603, 85.8564)
  line L143 (100.3205, 85.8564) -> (95.9904, 83.3564)
  line L144 (95.9904, 83.3564) -> (95.9904, 78.3564)
  line L145 (95.9904, 78.3564) -> (100.3205, 75.8564)
  line L146 (100.3205, 75.8564) -> (104.6506, 78.3564)
  line L147 (104.6506, 78.3564) -> (104.6506, 83.3564)
  line L148 (104.6506, 83.3564) -> (100.3205, 85.8564)
  line L149 (84.3301, 95.0885) -> (80, 92.5885)
  line L150 (80, 92.5885) -> (80, 87.5885)
  line L151 (80, 87.5885) -> (84.3301, 85.0885)
  line L152 (84.3301, 85.0885) -> (88.6603, 87.5885)
  line L153 (88.6603, 87.5885) -> (88.6603, 92.5885)
  line L154 (88.6603, 92.5885) -> (84.3301, 95.0885)
  line L155 (94.9904, 95.0885) -> (90.6603, 92.5885)
  line L156 (90.6603, 92.5885) -> (90.6603, 87.5885)
  line L157 (90.6603, 87.5885) -> (94.9904, 85.0885)
  line L158 (94.9904, 85.0885) -> (99.3205, 87.5885)
  line L159 (99.3205, 87.5885) -> (99.3205, 92.5885)
  line L160 (99.3205, 92.5885) -> (94.9904, 95.0885)
  line L161 (105.6506, 95.0885) -> (101.3205, 92.5885)
  line L162 (101.3205, 92.5885) -> (101.3205, 87.5885)
  line L163 (101.3205, 87.5885) -> (105.6506, 85.0885)
  line L164 (105.6506, 85.0885) -> (109.9808, 87.5885)
  line L165 (109.9808, 87.5885) -> (109.9808, 92.5885)
  line L166 (109.9808, 92.5885) -> (105.6506, 95.0885)
  line L167 (79, 104.3205) -> (74.6699, 101.8205)
  line L168 (74.6699, 101.8205) -> (74.6699, 96.8205)
  line L169 (74.6699, 96.8205) -> (79, 94.3205)
  line L170 (79, 94.3205) -> (83.3301, 96.8205)
  line L171 (83.3301, 96.8205) -> (83.3301, 101.8205)
  line L172 (83.3301, 101.8205) -> (79, 104.3205)
  line L173 (89.6603, 104.3205) -> (85.3301, 101.8205)
  line L174 (85.3301, 101.8205) -> (85.3301, 96.8205)
  line L175 (85.3301, 96.8205) -> (89.6603, 94.3205)
  line L176 (89.6603, 94.3205) -> (93.9904, 96.8205)
  line L177 (93.9904, 96.8205) -> (93.9904, 101.8205)
  line L178 (93.9904, 101.8205) -> (89.6603, 104.3205)
  line L179 (100.3205, 104.3205) -> (95.9904, 101.8205)
  line L180 (95.9904, 101.8205) -> (95.9904, 96.8205)
  line L181 (95.9904, 96.8205) -> (100.3205, 94.3205)
  line L182 (100.3205, 94.3205) -> (104.6506, 96.8205)
  line L183 (104.6506, 96.8205) -> (104.6506, 101.8205)
  line L184 (104.6506, 101.8205) -> (100.3205, 104.3205)
  line L185 (84.3301, 113.5526) -> (80, 111.0526)
  line L186 (80, 111.0526) -> (80, 106.0526)
  line L187 (80, 106.0526) -> (84.3301, 103.5526)
  line L188 (84.3301, 103.5526) -> (88.6603, 106.0526)
  line L189 (88.6603, 106.0526) -> (88.6603, 111.0526)
  line L190 (88.6603, 111.0526) -> (84.3301, 113.5526)
  line L191 (94.9904, 113.5526) -> (90.6603, 111.0526)
  line L192 (90.6603, 111.0526) -> (90.6603, 106.0526)
  line L193 (90.6603, 106.0526) -> (94.9904, 103.5526)
  line L194 (94.9904, 103.5526) -> (99.3205, 106.0526)
  line L195 (99.3205, 106.0526) -> (99.3205, 111.0526)
  line L196 (99.3205, 111.0526) -> (94.9904, 113.5526)
  line L197 (105.6506, 113.5526) -> (101.3205, 111.0526)
  line L198 (101.3205, 111.0526) -> (101.3205, 106.0526)
  line L199 (101.3205, 106.0526) -> (105.6506, 103.5526)
  line L200 (105.6506, 103.5526) -> (109.9808, 106.0526)
  line L201 (109.9808, 106.0526) -> (109.9808, 111.0526)
  line L202 (109.9808, 111.0526) -> (105.6506, 113.5526)
  line L203 (79, 122.7846) -> (74.6699, 120.2846)
  line L204 (74.6699, 120.2846) -> (74.6699, 115.2846)
  line L205 (74.6699, 115.2846) -> (79, 112.7846)
  line L206 (79, 112.7846) -> (83.3301, 115.2846)
  line L207 (83.3301, 115.2846) -> (83.3301, 120.2846)
  line L208 (83.3301, 120.2846) -> (79, 122.7846)
  line L209 (89.6603, 122.7846) -> (85.3301, 120.2846)
  line L210 (85.3301, 120.2846) -> (85.3301, 115.2846)
  line L211 (85.3301, 115.2846) -> (89.6603, 112.7846)
  line L212 (89.6603, 112.7846) -> (93.9904, 115.2846)
  line L213 (93.9904, 115.2846) -> (93.9904, 120.2846)
  line L214 (93.9904, 120.2846) -> (89.6603, 122.7846)
  line L215 (100.3205, 122.7846) -> (95.9904, 120.2846)
  line L216 (95.9904, 120.2846) -> (95.9904, 115.2846)
  line L217 (95.9904, 115.2846) -> (100.3205, 112.7846)
  line L218 (100.3205, 112.7846) -> (104.6506, 115.2846)
  line L219 (104.6506, 115.2846) -> (104.6506, 120.2846)
  line L220 (104.6506, 120.2846) -> (100.3205, 122.7846)
  line L221 (84.3301, 132.0167) -> (80, 129.5167)
  line L222 (80, 129.5167) -> (80, 124.5167)
  line L223 (80, 124.5167) -> (84.3301, 122.0167)
  line L224 (84.3301, 122.0167) -> (88.6603, 124.5167)
  line L225 (88.6603, 124.5167) -> (88.6603, 129.5167)
  line L226 (88.6603, 129.5167) -> (84.3301, 132.0167)
  line L227 (94.9904, 132.0167) -> (90.6603, 129.5167)
  line L228 (90.6603, 129.5167) -> (90.6603, 124.5167)
  line L229 (90.6603, 124.5167) -> (94.9904, 122.0167)
  line L230 (94.9904, 122.0167) -> (99.3205, 124.5167)
  line L231 (99.3205, 124.5167) -> (99.3205, 129.5167)
  line L232 (99.3205, 129.5167) -> (94.9904, 132.0167)
  line L233 (105.6506, 132.0167) -> (101.3205, 129.5167)
  line L234 (101.3205, 129.5167) -> (101.3205, 124.5167)
  line L235 (101.3205, 124.5167) -> (105.6506, 122.0167)
  line L236 (105.6506, 122.0167) -> (109.9808, 124.5167)
  line L237 (109.9808, 124.5167) -> (109.9808, 129.5167)
  line L238 (109.9808, 129.5167) -> (105.6506, 132.0167)
extrude "拉伸29" cut sketch "草图29" against normal blind 5 contours L5 L6 L7 L8 L9 L10 | L11 L12 L13 L14 L15 L16 | L17 L18 L19 L20 L21 L22 | L23 L24 L25 L26 L27 L28 | L29 L30 L31 L32 L33 L34 | L35 L36 L37 L38 L39 L40 | L41 L42 L43 L44 L45 L46 | L47 L48 L49 L50 L51 L52 | L53 L54 L55 L56 L57 L58 | L59 L60 L61 L62 L63 L64 | L65 L66 L67 L68 L69 L70 | L71 L72 L73 L74 L75 L76 | L77 L78 L79 L80 L81 L82 | L83 L84 L85 L86 L87 L88 | L89 L90 L91 L92 L93 L94 | L95 L96 L97 L98 L99 L100 | L101 L102 L103 L104 L105 L106 | L107 L108 L109 L110 L111 L112 | L113 L114 L115 L116 L117 L118 | L119 L120 L121 L122 L123 L124 | L125 L126 L127 L128 L129 L130 | L131 L132 L133 L134 L135 L136 | L137 L138 L139 L140 L141 L142 | L143 L144 L145 L146 L147 L148 | L149 L150 L151 L152 L153 L154 | L155 L156 L157 L158 L159 L160 | L161 L162 L163 L164 L165 L166 | L167 L168 L169 L170 L171 L172 | L173 L174 L175 L176 L177 L178 | L179 L180 L181 L182 L183 L184 | L185 L186 L187 L188 L189 L190 | L191 L192 L193 L194 L195 L196 | L197 L198 L199 L200 L201 L202 | L203 L204 L205 L206 L207 L208 | L209 L210 L211 L212 L213 L214 | L215 L216 L217 L218 L219 L220 | L221 L222 L223 L224 L225 L226 | L227 L228 L229 L230 L231 L232 | L233 L234 L235 L236 L237 L238 bodies 1
equation "d29 = '胶带160'"
equation "d49 = '大钳95 '"
equation "d58 = '小钳95'"
equation "d64 = '杂物140'"
equation "d69 = '电工钳95 '"
equation "d85 = '卡尺140'"
equation "d87 = '扳手80 '"
equation "d89 = '铲子70'"
equation "d91 = '电子尺60'"
equation "d120 = '剪刀65'"
equation "d123 = '小刀70'"
equation "d126 = '电笔70'"
equation "d137 = '杂物60 '"
equation "d330 = -( 3.00 mm )"
equation "d344 = -( 5.00 mm )"
equation "d346 = -( 5.00 mm )"
